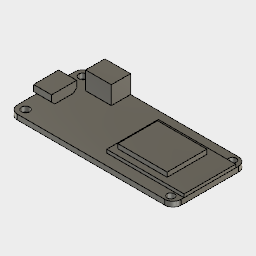
Feather Huzzah v1 (Autodesk Fusion 360 design; units mm, degrees)
Autodesk Fusion 360 part; units mm, degrees
note: some values were not read from the file. Set by a fixed rule: which sketch regions a step uses.
sketch "PCB" plane through (0, 0, 0) normal (0, 0, 1) x (1, 0, 0)
  line L0 (0, 0) -> (50.8, 0)
  line L1 (50.8, 0) -> (50.8, -22.86)
  line L2 (50.8, -22.86) -> (0, -22.86)
  line L3 (0, -22.86) -> (0, 0)
  circle A0 centre (2.54, -20.32) radius 1.27
  circle A1 centre (2.54, -2.54) radius 1.27
  circle A2 centre (48.26, -21.0185) radius 1.145
  circle A3 centre (48.26, -1.905) radius 1.145
  dimension "d1" = 50.8
  dimension "d2" = 22.86
  dimension "d3" = 2.54
  dimension "d4" = 2.54
  dimension "d5" = 2.54
  dimension "d6" = 2.54
  dimension "d7" = 20.32
  dimension "d8" = 2.54
  dimension "d9" = 2.29
  dimension "d10" = 48.26
  dimension "d11" = 1.8415
  dimension "d12" = 2.29
  dimension "d13" = 20.955
  dimension "d14" = 48.26
  measures "d1" distance of L0.start L0.end
  measures "d2" distance of L0.start L2.end
  measures "d3" diameter of A0
  measures "d4" distance of L3 A0.centre
  measures "d5" distance of L2 A0.centre
  measures "d6" diameter of A1
  measures "d7" distance of L2 A1.centre
  measures "d8" distance of L3 A1.centre
  measures "d9" diameter of A2
  measures "d10" distance of L3 A2.centre
  measures "d11" distance of L2 A2.centre
  measures "d12" diameter of A3
  measures "d13" distance of L2 A3.centre
  measures "d14" distance of L3 A3.centre
extrude "Extrude1" add sketch "PCB" along normal blind 1.6 makes body 1
fillet "Fillet1" radius 2.54 4 edges at (0, -22.86, 0.8) (50.8, -22.86, 0.8) (50.8, 0, 0.8) (0, 0, 0.8) on bodies 1
sketch "usb" plane through (0, 0, 1.6) normal (0, 0, 1) x (-1, 0, 0)
  circle A0 centre (-2.54, 20.32) radius 1.27
  circle A1 centre (-2.54, 2.54) radius 1.27
  circle A2 centre (-48.26, 21.0185) radius 1.145
  circle A3 centre (-48.26, 1.905) radius 1.145
  arc A4 (-2.54, 0) -> (0, 2.54) centre (-2.54, 2.54) ccw
  line L0 (0, 2.54) -> (0, 20.32)
  arc A5 (0, 20.32) -> (-2.54, 22.86) centre (-2.54, 20.32) ccw
  line L1 (-2.54, 22.86) -> (-48.26, 22.86)
  arc A6 (-48.26, 22.86) -> (-50.8, 20.32) centre (-48.26, 20.32) ccw
  line L2 (-50.8, 20.32) -> (-50.8, 2.54)
  arc A7 (-50.8, 2.54) -> (-48.26, 0) centre (-48.26, 2.54) ccw
  line L3 (-48.26, 0) -> (-2.54, 0)
  line L4 (0, 11.43) -> (-50.8, 11.43) construction
  line L5 (0, 15.33) -> (-5.6, 15.33)
  line L6 (-5.6, 15.33) -> (-5.6, 7.53)
  line L7 (-5.6, 7.53) -> (0, 7.53)
  line L8 (0, 7.53) -> (0, 15.33)
  line L9 (0, 15.33) -> (-5.6, 7.53) construction
  line L10 (-5.6, 15.33) -> (0, 7.53) construction
  point P0 (-2.8, 11.43)
  dimension "d18" = 7.8
  dimension "d19" = 5.6
  measures "d18" distance of L5.end L6.end
  measures "d19" distance of L6.end L7.end
extrude "Extrude2" add sketch "usb" along normal blind 2.95 separate body contours L0 L5 L6 L7 L8 makes body 2
chamfer "Chamfer1" distance 1 angle 45 2 edges at (2.8, -7.53, 1.6) (2.8, -15.33, 1.6) on bodies 2
sketch "modules" plane through (0, 0, 1.6) normal (0, 0, 1) x (-1, 0, 0)
  circle A0 centre (-2.54, 20.32) radius 1.27
  circle A1 centre (-2.54, 2.54) radius 1.27
  circle A2 centre (-48.26, 21.0185) radius 1.145
  circle A3 centre (-48.26, 1.905) radius 1.145
  arc A4 (-2.54, 0) -> (0, 2.54) centre (-2.54, 2.54) ccw
  line L0 (0, 2.54) -> (0, 20.32)
  arc A5 (0, 20.32) -> (-2.54, 22.86) centre (-2.54, 20.32) ccw
  line L1 (-2.54, 22.86) -> (-48.26, 22.86)
  arc A6 (-48.26, 22.86) -> (-50.8, 20.32) centre (-48.26, 20.32) ccw
  line L2 (-50.8, 20.32) -> (-50.8, 2.54)
  arc A7 (-50.8, 2.54) -> (-48.26, 0) centre (-48.26, 2.54) ccw
  line L3 (-48.26, 0) -> (-2.54, 0)
  line L4 (-50.8, 11.43) -> (0, 11.43) construction
  line L5 (-26.8, 19.43) -> (-50.8, 19.43)
  line L6 (-50.8, 19.43) -> (-50.8, 3.43)
  line L7 (-50.8, 3.43) -> (-26.8, 3.43)
  line L8 (-26.8, 3.43) -> (-26.8, 19.43)
  line L9 (-26.8, 19.43) -> (-50.8, 3.43) construction
  line L10 (-50.8, 19.43) -> (-26.8, 3.43) construction
  line L11 (-28.4, 17.58) -> (-43.7, 17.58)
  line L12 (-43.7, 17.58) -> (-43.7, 5.28)
  line L13 (-43.7, 5.28) -> (-28.4, 5.28)
  line L14 (-28.4, 5.28) -> (-28.4, 17.58)
  line L15 (-28.4, 17.58) -> (-43.7, 5.28) construction
  line L16 (-43.7, 17.58) -> (-28.4, 5.28) construction
  point P0 (-38.8, 11.43)
  point P1 (-36.05, 11.43)
  dimension "d23" = 24
  dimension "d24" = 16
  dimension "d25" = 15.3
  dimension "d26" = 12.3
  dimension "d32" = 1.6
  measures "d23" distance of L6.end L7.end
  measures "d24" distance of L5.end L6.end
  measures "d25" distance of L12.end L13.end
  measures "d26" distance of L11.end L12.end
  measures "d32" distance of L8 L14
extrude "Extrude3" add sketch "modules" along normal blind 1 separate body contours L2 L5 L6 L7 L8 | L11 L12 L13 L14 makes body 3
extrude "Extrude4" add sketch "modules" along normal blind 2.4 and the other way blind -1 separate body contours L11 L12 L13 L14 makes body 4
sketch "JST" plane through (0, 0, 1.6) normal (0, 0, 1) x (-1, 0, 0)
  circle A0 centre (-2.54, 20.32) radius 1.27
  circle A1 centre (-2.54, 2.54) radius 1.27
  circle A2 centre (-48.26, 21.0185) radius 1.145
  circle A3 centre (-48.26, 1.905) radius 1.145
  arc A4 (-2.54, 0) -> (0, 2.54) centre (-2.54, 2.54) ccw
  line L0 (0, 2.54) -> (0, 20.32)
  arc A5 (0, 20.32) -> (-2.54, 22.86) centre (-2.54, 20.32) ccw
  line L1 (-2.54, 22.86) -> (-48.26, 22.86)
  arc A6 (-48.26, 22.86) -> (-50.8, 20.32) centre (-48.26, 20.32) ccw
  line L2 (-50.8, 20.32) -> (-50.8, 2.54)
  arc A7 (-50.8, 2.54) -> (-48.26, 0) centre (-48.26, 2.54) ccw
  line L3 (-48.26, 0) -> (-2.54, 0)
  line L4 (-6.8, 0) -> (-14.8, 0)
  line L5 (-14.8, 0) -> (-14.8, 6)
  line L6 (-14.8, 6) -> (-6.8, 6)
  line L7 (-6.8, 6) -> (-6.8, 0)
  line L8 (-10.8, 0) -> (-10.8, 6) construction
  dimension "d33" = 8
  dimension "d34" = 6
  dimension "d35" = 10.8
  measures "d33" distance of L4.start L4.end
  measures "d34" distance of L4.start L6.end
  measures "d35" distance of L0 L8
extrude "Extrude5" add sketch "JST" along normal blind 5.6 separate body contours L3 L4 L5 L6 L7 makes body 5
named bodies: "Huzzah PCB", "usb", "wifi pcb", "wifi mod", "JST"
